Autodesk Inventor part; units mm, degrees
note: some values were not read from the file. Chosen so that the rebuilt part matches the saved one: direction of "Hole2".
(part 9 of 20)
  ellipse E68 centre (-104.430172, -37.80624) end of major axis (-105.229069, -37.764253) minor radius 0.002573 (-104.767308, -37.786185) -> (-104.757911, -37.791366) ccw
  line L116 (-105.229069, -37.764253) -> (-105.124102, -35.76702)
  line L117 (-102.853693, -35.883206) -> (-102.767428, -34.241823)
  line L118 (-103.727851, -35.778425) -> (-103.715482, -35.543073)
  ellipse E69 centre (-104.430172, -37.80624) end of major axis (-104.929483, -37.779998) minor radius 0.001608 (-104.765064, -37.787445) -> (-104.760245, -37.790101) ccw
  line L119 (-91.805643, -35.801391) -> (-92.357488, -33.197777)
  ellipse E70 centre (-90.362382, -35.950654) end of major axis (-88.992808, -35.660368) minor radius 0.211294 (-90.910001, -35.866075) -> (-90.933885, -35.8727) ccw
  line L120 (-90.98715, -35.502085) -> (-90.910001, -35.866075)
  line L121 (-91.937822, -36.388821) -> (-91.841267, -36.339714)
  line L122 (-90.910001, -35.866075) -> (-90.833464, -35.827148)
  line L123 (-91.937822, -36.388821) -> (-90.397989, -36.081252)
  ellipse E71 centre (-90.362382, -35.950654) end of major axis (-89.579768, -35.784776) minor radius 0.120739 (-90.397989, -36.081252) -> (-89.740826, -35.747021) ccw
  line L124 (-89.740826, -35.747021) -> (-90.657006, -35.748201)
  line L125 (-91.73285, -37.355883) -> (-91.937822, -36.388821)
  ellipse E72 centre (-89.952438, -37.884777) end of major axis (-90.735052, -38.050655) minor radius 0.120739 (-90.64361, -38.085759) -> (-89.235774, -37.786185) ccw
  line L126 (-89.578101, -35.792644) -> (-89.579768, -35.784776)
  line L127 (-91.937822, -36.388821) -> (-92.608968, -33.222344)
  line L128 (-91.73285, -37.355883) -> (-92.054619, -37.098206)
  ellipse E73 centre (-91.737472, -36.936906) end of major axis (-92.531076, -36.371583) minor radius 0.319988 (-92.547253, -36.492324) -> (-92.054619, -37.098206) ccw
  line L129 (-92.547253, -36.492324) -> (-93.874248, -30.231533)
  line L130 (-91.73285, -37.355883) -> (-90.193017, -37.048314)
  line L131 (-89.325137, -35.77526) -> (-89.388482, -35.213586)
  line L132 (-88.451238, -35.605729) -> (-88.440782, -35.698444)
  line L133 (-88.870762, -35.923384) -> (-88.001691, -35.82361)
  ellipse E74 centre (-87.925465, -35.832087) end of major axis (-87.130505, -35.742432) minor radius 0.01704 (-87.143191, -35.740852) -> (-88.001691, -35.82361) ccw
  ellipse E75 centre (-87.70138, -37.819037) end of major axis (-88.496341, -37.908691) minor radius 0.01704 (-86.979081, -37.730452) -> (-88.427677, -37.893938) ccw
  line L134 (-89.589644, -35.734525) -> (-89.646842, -35.227355)
  ellipse E76 centre (-89.482855, -22.022782) end of major axis (-87.406021, -21.788561) minor radius 0.044517 (-87.474249, -21.78497) -> (-87.899556, -21.815311) ccw
  ellipse E77 centre (-89.382017, -22.91691) end of major axis (-87.305183, -22.682688) minor radius 0.044517 (-87.376049, -22.679181) -> (-87.795125, -22.709125) ccw
  ellipse E78 centre (-87.813423, -36.825562) end of major axis (-88.608383, -36.915216) minor radius 0.01704 (-87.889648, -36.817085) -> (-88.582568, -36.90793) ccw
  line L135 (-88.81819, -36.923686) -> (-87.889648, -36.817085)
  ellipse E79 centre (-87.70138, -37.819037) end of major axis (-88.198231, -37.875071) minor radius 0.01065 (-87.22685, -37.762368) -> (-88.190637, -37.872322) ccw
  line L136 (-95.422117, -34.951561) -> (-95.372421, -34.494843)
  line L137 (-93.334624, -36.847285) -> (-94.485298, -36.84101)
  line L138 (-94.326748, -37.421303) -> (-93.014694, -37.428457)
  line L139 (-93.014694, -37.428457) -> (-92.908579, -37.255208)
  ellipse E80 centre (-93.582228, -37.251534) end of major axis (-92.87059, -37.067245) minor radius 0.371687 (-93.186534, -36.858933) -> (-93.334624, -36.847285) ccw
  ellipse E81 centre (-93.582228, -37.251534) end of major axis (-92.87059, -37.067245) minor radius 0.371687 (-92.908579, -37.255208) -> (-92.903906, -37.247372) ccw
  ellipse E82 centre (-94.728774, -37.966559) end of major axis (-93.933469, -38.053098) minor radius 0.273562 (-94.113945, -38.200163) -> (-93.998225, -38.145751) ccw
  line L140 (-98.417199, -34.951561) -> (-98.466895, -34.494843)
  ellipse E83 centre (-100.277081, -37.276138) end of major axis (-99.56931, -37.369327) minor radius 0.400382 (-100.444305, -36.869727) -> (-100.966797, -37.309126) ccw
  line L141 (-100.985403, -37.237624) -> (-101.000691, -37.09713)
  line L142 (-99.513466, -36.825206) -> (-100.444305, -36.869727)
  line L143 (-100.966797, -37.309126) -> (-100.895129, -37.483302)
  line L144 (-100.895129, -37.483302) -> (-99.67736, -37.425058)
  ellipse E84 centre (-99.274308, -37.966559) end of major axis (-100.069614, -38.053098) minor radius 0.273562 (-100.004857, -38.145751) -> (-99.889137, -38.200163) ccw
  ellipse E85 centre (-106.077617, -35.832087) end of major axis (-106.872577, -35.742432) minor radius 0.01704 (-106.083328, -35.814295) -> (-106.859892, -35.740852) ccw
  line L145 (-106.083328, -35.814295) -> (-105.132213, -35.921364)
  ellipse E86 centre (-106.301702, -37.819037) end of major axis (-107.096662, -37.729383) minor radius 0.01704 (-105.575405, -37.893938) -> (-107.024001, -37.730452) ccw
  line L146 (-104.489789, -35.736592) -> (-104.431907, -35.22335)
  ellipse E87 centre (-104.520227, -22.022782) end of major axis (-106.597061, -21.788561) minor radius 0.044517 (-106.103527, -21.815311) -> (-106.597061, -21.788561) ccw
  ellipse E88 centre (-104.621065, -22.91691) end of major axis (-106.697899, -22.682688) minor radius 0.044517 (-106.207957, -22.709125) -> (-106.627033, -22.679181) ccw
  line L147 (-106.195371, -36.80777) -> (-105.184779, -36.921534)
  ellipse E89 centre (-106.189659, -36.825562) end of major axis (-105.394699, -36.915216) minor radius 0.01704 (-105.420514, -36.90793) -> (-106.195371, -36.80777) ccw
  ellipse E90 centre (-106.301702, -37.819037) end of major axis (-106.798552, -37.763003) minor radius 0.01065 (-105.858125, -37.873868) -> (-106.750481, -37.773047) ccw
  line L148 (-103.182559, -35.813202) -> (-104.167244, -35.750402)
  ellipse E91 centre (-103.6407, -35.950654) end of major axis (-104.423314, -35.784776) minor radius 0.120739 (-104.167244, -35.750402) -> (-103.745321, -36.051258) ccw
  line L149 (-103.745321, -36.051258) -> (-102.217715, -36.399788)
  line L150 (-102.217715, -36.399788) -> (-102.422687, -37.36685)
  ellipse E92 centre (-104.050644, -37.884777) end of major axis (-104.833258, -37.718899) minor radius 0.120739 (-104.767308, -37.786185) -> (-103.359472, -38.085759) ccw
  line L151 (-104.424982, -35.792644) -> (-104.423314, -35.784776)
  line L152 (-102.250485, -36.376421) -> (-102.217715, -36.399788)
  line L153 (-102.217715, -36.399788) -> (-101.541613, -33.209926)
  ellipse E93 centre (-102.284453, -36.9758) end of major axis (-101.472148, -36.416877) minor radius 0.235923 (-102.080832, -37.120994) -> (-101.472427, -36.509437) ccw
  line L154 (-101.404603, -36.200633) -> (-100.152123, -30.291408)
  line L155 (-102.080832, -37.120994) -> (-102.422687, -37.36685)
  line L156 (-103.950293, -37.01832) -> (-102.422687, -37.36685)
  line L157 (-91.05411, -35.879044) -> (-91.076939, -35.444665)
  line L158 (-90.230803, -35.465481) -> (-90.215974, -35.747633)
  line L159 (-91.29938, -35.891986) -> (-89.730041, -35.809177)
  ellipse E94 centre (-89.677878, -35.809007) end of major axis (-88.87898, -35.76702) minor radius 0.002573 (-88.87898, -35.76702) -> (-89.730041, -35.809177) ccw
  line L160 (-91.296789, -35.941292) -> (-91.29938, -35.891986)
  ellipse E95 centre (-89.57291, -37.80624) end of major axis (-88.774013, -37.764253) minor radius 0.002573 (-89.245172, -37.791366) -> (-89.235774, -37.786185) ccw
  line L161 (-88.774013, -37.764253) -> (-88.87898, -35.76702)
  line L162 (-89.970222, -35.743864) -> (-89.985769, -35.448055)
  line L163 (-91.29938, -35.891986) -> (-91.385523, -34.252933)
  ellipse E96 centre (-89.57291, -37.80624) end of major axis (-89.073599, -37.779998) minor radius 0.001608 (-89.242837, -37.790101) -> (-89.238018, -37.787445) ccw
  line L164 (-88.579416, -35.694157) -> (-88.575478, -35.616282)
  line L165 (-87.658407, -35.518527) -> (-87.66871, -35.722319)
  line L166 (-88.844477, -35.685961) -> (-87.279448, -35.734356)
  ellipse E97 centre (-87.199512, -35.880709) end of major axis (-86.400533, -35.921103) minor radius 0.142983 (-86.400533, -35.921103) -> (-86.916832, -35.760642) ccw
  line L167 (-88.846734, -35.730605) -> (-88.844477, -35.685961)
  ellipse E98 centre (-87.298871, -37.845996) end of major axis (-86.499891, -37.88639) minor radius 0.142983 (-86.638988, -37.959011) -> (-86.979081, -37.730452) ccw
  line L168 (-86.499891, -37.88639) -> (-86.400533, -35.921103)
  line L169 (-87.403649, -35.730515) -> (-87.391234, -35.48496)
  line L170 (-88.844477, -35.685961) -> (-88.834557, -35.489748)
  line L171 (-88.754671, -33.90963) -> (-88.741991, -33.658819)
  ellipse E99 centre (-86.508969, -22.221966) end of major axis (-84.421635, -22.327495) minor radius 0.373543 (-84.421635, -22.327495) -> (-85.857037, -21.898574) ccw
  ellipse E100 centre (-86.553681, -23.106345) end of major axis (-84.466347, -23.211874) minor radius 0.373543 (-84.855794, -23.407002) -> (-85.889952, -22.784232) ccw
  line L172 (-84.421635, -22.327495) -> (-84.466347, -23.211874)
  ellipse E101 centre (-86.553681, -23.106345) end of major axis (-85.055594, -23.182084) minor radius 0.268093 (-85.19814, -23.286981) -> (-87.773888, -22.890892) ccw
  ellipse E102 centre (-87.298871, -37.845996) end of major axis (-86.799509, -37.871242) minor radius 0.089364 (-87.113287, -37.938145) -> (-87.283323, -37.757325) ccw
  line L173 (-92.998906, -37.402681) -> (-92.513899, -37.499993)
  line L174 (-92.513899, -37.499993) -> (-92.504619, -37.487523)
  ellipse E103 centre (-94.353837, -37.924209) end of major axis (-93.580574, -38.129305) minor radius 0.142054 (-93.998225, -38.145751) -> (-93.580574, -38.129305) ccw
  line L175 (-93.580574, -38.129305) -> (-93.394136, -37.426388)
  line L176 (-97.450158, -34.951561) -> (-97.421801, -34.494843)
  line L177 (-105.395973, -36.91016) -> (-105.187286, -36.969239)
  ellipse E104 centre (-105.630208, -36.995775) end of major axis (-106.398891, -36.77413) minor radius 0.14613 (-105.188594, -36.994129) -> (-105.420514, -36.90793) ccw
  ellipse E105 centre (-105.902602, -37.940463) end of major axis (-105.422175, -38.078991) minor radius 0.091331 (-105.743445, -38.074276) -> (-105.879328, -37.852122) ccw
  ellipse E106 centre (-105.902602, -37.940463) end of major axis (-105.133919, -38.162107) minor radius 0.14613 (-105.634452, -38.157355) -> (-105.575405, -37.893938) ccw
  line L178 (-105.133919, -38.162107) -> (-105.022824, -37.776821)
  ellipse E107 centre (-102.93673, -36.106911) end of major axis (-103.682535, -35.817472) minor radius 0.002457 (-103.628417, -35.837492) -> (-103.682535, -35.817472) ccw
  ellipse E108 centre (-102.93673, -36.106911) end of major axis (-102.190924, -36.39635) minor radius 0.002457 (-103.612298, -35.843617) -> (-103.614549, -35.842761) ccw
  line L179 (-101.551416, -36.641447) -> (-101.540632, -36.645629)
  line L180 (-101.540632, -36.645629) -> (-101.902428, -37.577881)
  ellipse E109 centre (-103.660323, -37.971415) end of major axis (-102.914518, -38.260854) minor radius 0.002457 (-103.369821, -38.086582) -> (-103.359472, -38.085759) ccw
  line L181 (-103.68619, -35.82689) -> (-103.682535, -35.817472)
  line L182 (-102.914518, -38.260854) -> (-102.55578, -37.336484)
  line L183 (-101.540632, -36.645629) -> (-101.524884, -36.605051)
  line L184 (-101.452389, -36.418253) -> (-99.538445, -31.486535)
  ellipse E110 centre (-101.752662, -37.31671) end of major axis (-100.860337, -36.923935) minor radius 0.168714 (-101.530862, -37.400618) -> (-100.861799, -36.955978) ccw
  line L185 (-100.861799, -36.955978) -> (-99.208221, -32.695154)
  line L186 (-101.530862, -37.400618) -> (-101.902428, -37.577881)
  line L187 (-101.902428, -37.577881) -> (-102.517352, -37.345251)
  line L188 (-102.480897, -37.353569) -> (-101.902428, -37.577881)
  ellipse E111 centre (-103.660323, -37.971415) end of major axis (-103.194195, -38.152314) minor radius 0.001536 (-103.367332, -38.086401) -> (-103.361886, -38.085968) ccw
  line L189 (-91.613539, -36.134298) -> (-90.335363, -35.889978)
  ellipse E112 centre (-90.284268, -35.882488) end of major axis (-89.498467, -35.732431) minor radius 0.002231 (-90.135583, -35.851865) -> (-90.335363, -35.889978) ccw
  ellipse E113 centre (-90.284268, -35.882488) end of major axis (-89.498467, -35.732431) minor radius 0.002231 (-89.498467, -35.732431) -> (-89.980553, -35.822396) ccw
  line L190 (-89.497225, -35.738934) -> (-89.498467, -35.732431)
  line L191 (-88.873766, -35.866229) -> (-87.933724, -35.761265)
  ellipse E114 centre (-89.104953, -23.113274) end of major axis (-87.612095, -22.967065) minor radius 0.24157 (-87.677538, -22.90597) -> (-87.775629, -22.875994) ccw
  ellipse E115 centre (-89.104953, -23.113274) end of major axis (-87.024905, -22.909556) minor radius 0.336587 (-87.098371, -22.83267) -> (-87.104345, -22.829762) ccw
  ellipse E116 centre (-87.66195, -37.846982) end of major axis (-88.15957, -37.895718) minor radius 0.080523 (-88.095363, -37.848555) -> (-88.145676, -37.874094) ccw
  ellipse E117 centre (-87.66195, -37.846982) end of major axis (-87.164331, -37.798246) minor radius 0.080523 (-87.174632, -37.784081) -> (-87.288761, -37.757867) ccw
  ellipse E118 centre (-103.712607, -35.91066) end of major axis (-102.927191, -36.062721) minor radius 0.086818 (-103.766394, -35.812171) -> (-104.360228, -35.736765) ccw
  line L192 (-103.766394, -35.812171) -> (-103.588186, -35.844875)
  line L193 (-91.006251, -36.071199) -> (-90.764705, -35.999517)
  ellipse E119 centre (-90.71868, -35.988107) end of major axis (-89.951703, -35.76063) minor radius 0.002152 (-90.57202, -35.942407) -> (-90.764705, -35.999517) ccw
  ellipse E120 centre (-90.71868, -35.988107) end of major axis (-89.951703, -35.76063) minor radius 0.002152 (-90.500776, -35.921328) -> (-90.503346, -35.922088) ccw
  ellipse E121 centre (-90.71868, -35.988107) end of major axis (-89.951703, -35.76063) minor radius 0.002152 (-89.952246, -35.760708) -> (-90.205619, -35.834272) ccw
  line L194 (-91.987497, -37.405497) -> (-92.086263, -37.07249)
  line L195 (-94.014167, -29.871815) -> (-94.02426, -29.874754)
  line L196 (-93.270796, -33.078635) -> (-94.118611, -30.22008)
  line L197 (-91.976236, -37.402218) -> (-91.987497, -37.405497)
  line L198 (-91.987497, -37.405497) -> (-92.05118, -37.365553)
  line L199 (-91.987497, -37.405497) -> (-91.756499, -37.336945)
  line L200 (-88.415292, -35.841908) -> (-88.397731, -35.838079)
  ellipse E122 centre (-88.323123, -35.953616) end of major axis (-87.539825, -35.791) minor radius 0.128538 (-88.161995, -35.792662) -> (-88.397731, -35.838079) ccw
  line L201 (-88.817348, -36.939713) -> (-88.754142, -36.925932)
  ellipse E123 centre (-87.921864, -37.88642) end of major axis (-88.411426, -37.988055) minor radius 0.080336 (-88.12131, -37.851814) -> (-88.276833, -38.014639) ccw
  ellipse E124 centre (-106.609775, -35.858739) end of major axis (-107.409757, -35.864011) minor radius 0.125799 (-106.589584, -35.732848) -> (-107.409757, -35.864011) ccw
  line L202 (-106.589584, -35.732848) -> (-105.874946, -35.731093)
  line L203 (-105.036889, -35.729035) -> (-105.015254, -35.728981)
  line L204 (-105.015254, -35.728981) -> (-105.015061, -35.758236)
  ellipse E125 centre (-106.59676, -37.833815) end of major axis (-107.396743, -37.839086) minor radius 0.125799 (-106.311855, -37.714431) -> (-106.576569, -37.707924) ccw
  line L205 (-105.015254, -35.728981) -> (-105.018797, -35.191274)
  line L206 (-105.025415, -34.186857) -> (-105.028812, -33.671406)
  ellipse E126 centre (-106.700226, -22.131966) end of major axis (-108.790181, -22.145737) minor radius 0.328649 (-106.862517, -21.805345) -> (-107.891271, -21.869557) ccw
  ellipse E127 centre (-106.69437, -23.02075) end of major axis (-108.784324, -23.034521) minor radius 0.328649 (-106.93899, -22.695925) -> (-107.877588, -22.757441) ccw
  ellipse E128 centre (-106.69437, -23.02075) end of major axis (-108.194337, -23.030633) minor radius 0.235872 (-106.217877, -22.794028) -> (-108.191997, -23.043547) ccw
  ellipse E129 centre (-106.59676, -37.833815) end of major axis (-107.096749, -37.837109) minor radius 0.078624 (-106.71236, -37.758062) -> (-106.891764, -37.899192) ccw
  ellipse E130 centre (-104.183501, -35.818698) end of major axis (-104.980671, -35.751457) minor radius 0.002201 (-104.267264, -35.809437) -> (-104.980671, -35.751457) ccw
  line L207 (-104.981419, -35.760336) -> (-104.980671, -35.751457)
  line L208 (-91.61255, -36.134109) -> (-92.161706, -33.174903)
  line L209 (-91.833694, -36.261711) -> (-91.607996, -36.175948)
  line L210 (-91.833694, -36.261711) -> (-90.286036, -35.982923)
  ellipse E131 centre (-90.257477, -35.898912) end of major axis (-89.470906, -35.752944) minor radius 0.077504 (-90.286036, -35.982923) -> (-89.630523, -35.736086) ccw
  ellipse E132 centre (-90.257477, -35.898912) end of major axis (-91.044047, -36.044881) minor radius 0.077504 (-89.632187, -35.736173) -> (-89.637416, -35.736455) ccw
  line L211 (-89.637416, -35.736455) -> (-89.681705, -35.738912)
  line L212 (-91.827408, -36.295579) -> (-91.833694, -36.261711)
  line L213 (-89.464627, -35.786781) -> (-89.470906, -35.752944)
  line L214 (-91.833694, -36.261711) -> (-92.093462, -34.861913)
  line L215 (-89.25094, -35.769186) -> (-89.305654, -35.209109)
  line L216 (-88.872594, -35.888539) -> (-87.92125, -35.79153)
  ellipse E133 centre (-87.858242, -35.831451) end of major axis (-87.062032, -35.753669) minor radius 0.045982 (-87.119951, -35.742267) -> (-87.92125, -35.79153) ccw
  line L217 (-89.505008, -35.733389) -> (-89.554918, -35.222487)
  ellipse E134 centre (-89.207472, -22.020177) end of major axis (-87.127374, -21.816972) minor radius 0.120129 (-87.140565, -21.805345) -> (-87.901453, -21.799074) ccw
  ellipse E135 centre (-89.120111, -22.914432) end of major axis (-87.040013, -22.711227) minor radius 0.120129 (-87.064092, -22.695925) -> (-87.308637, -22.678729) ccw
  ellipse E136 centre (-89.120111, -22.914432) end of major axis (-87.627218, -22.768591) minor radius 0.086217 (-87.781875, -22.822534) -> (-87.790867, -22.745575) ccw
  ellipse E137 centre (-87.664108, -37.818684) end of major axis (-87.166477, -37.77007) minor radius 0.028739 (-87.20767, -37.762739) -> (-87.224132, -37.762354) ccw
  line L218 (-104.713483, -35.208237) -> (-104.768154, -35.767882)
  ellipse E138 centre (-106.144841, -35.831451) end of major axis (-106.94105, -35.753669) minor radius 0.045982 (-106.128174, -35.786883) -> (-106.883131, -35.742267) ccw
  line L219 (-106.128174, -35.786883) -> (-105.130316, -35.885252)
  ellipse E139 centre (-104.795611, -22.020177) end of major axis (-106.875708, -21.816972) minor radius 0.120129 (-106.101629, -21.799074) -> (-106.862517, -21.805345) ccw
  ellipse E140 centre (-104.882971, -22.914432) end of major axis (-106.963069, -22.711227) minor radius 0.120129 (-106.694445, -22.678729) -> (-106.93899, -22.695925) ccw
  ellipse E141 centre (-104.882971, -22.914432) end of major axis (-106.375864, -22.768591) minor radius 0.086217 (-106.212215, -22.745575) -> (-106.221207, -22.822534) ccw
  ellipse E142 centre (-106.338974, -37.818684) end of major axis (-105.841343, -37.867298) minor radius 0.028739 (-105.860305, -37.873186) -> (-105.881624, -37.851833) ccw
  ellipse E143 centre (-106.338974, -37.818684) end of major axis (-106.836605, -37.77007) minor radius 0.028739 (-106.618921, -37.767554) -> (-106.813201, -37.781264) ccw
  line L220 (-101.888103, -33.169443) -> (-102.432316, -36.102017)
  ellipse E144 centre (-103.745605, -35.898912) end of major axis (-104.532176, -35.752944) minor radius 0.077504 (-104.360228, -35.736765) -> (-103.821607, -35.963391) ccw
  line L221 (-103.821607, -35.963391) -> (-102.343144, -36.249471)
  line L222 (-104.538455, -35.786781) -> (-104.532176, -35.752944)
  line L223 (-91.426481, -35.952249) -> (-89.859121, -35.819828)
  ellipse E145 centre (-89.819581, -35.818698) end of major axis (-89.022412, -35.751457) minor radius 0.002201 (-89.737454, -35.809574) -> (-89.859121, -35.819828) ccw
  ellipse E146 centre (-89.819581, -35.818698) end of major axis (-89.022412, -35.751457) minor radius 0.002201 (-89.022412, -35.751457) -> (-89.737257, -35.809558) ccw
  line L224 (-91.414337, -36.096221) -> (-91.426481, -35.952249)
  line L225 (-89.021663, -35.760336) -> (-89.022412, -35.751457)
  line L226 (-91.426481, -35.952249) -> (-91.57069, -34.242604)
  line L227 (-91.663147, -33.146486) -> (-91.665639, -33.116944)
  line L228 (-87.900207, -35.546912) -> (-87.901315, -35.715126)
  line L229 (-89.02939, -35.743523) -> (-87.460048, -35.732948)
  ellipse E147 centre (-87.393307, -35.858739) end of major axis (-86.593325, -35.864011) minor radius 0.125799 (-86.959772, -35.755799) -> (-87.460048, -35.732948) ccw
  line L230 (-89.029444, -35.751758) -> (-89.02939, -35.743523)
  line L231 (-89.02939, -35.743523) -> (-89.025766, -35.193642)
  line L232 (-89.019145, -34.188784) -> (-89.013946, -33.399804)
  ellipse E148 centre (-87.302856, -22.131966) end of major axis (-89.392811, -22.118194) minor radius 0.328649 (-86.111811, -21.869557) -> (-87.140565, -21.805345) ccw
  ellipse E149 centre (-87.308712, -23.02075) end of major axis (-89.398667, -23.006978) minor radius 0.328649 (-86.125494, -22.757441) -> (-87.064092, -22.695925) ccw
  ellipse E150 centre (-87.308712, -23.02075) end of major axis (-85.808745, -23.030633) minor radius 0.235872 (-85.826668, -23.06663) -> (-87.785206, -22.794028) ccw
  ellipse E151 centre (-87.399815, -36.846277) end of major axis (-88.199797, -36.841005) minor radius 0.125799 (-87.466556, -36.720485) -> (-87.787907, -36.733777) ccw
  ellipse E152 centre (-87.406322, -37.833815) end of major axis (-86.906333, -37.837109) minor radius 0.078624 (-87.053751, -37.780331) -> (-87.290722, -37.758062) ccw
  line L233 (-105.197035, -36.931057) -> (-105.185407, -36.933478)
  ellipse E153 centre (-106.081218, -37.88642) end of major axis (-105.591656, -37.988055) minor radius 0.080336 (-105.726249, -38.014639) -> (-105.881772, -37.851814) ccw
  ellipse E154 centre (-103.284402, -35.988107) end of major axis (-104.051379, -35.76063) minor radius 0.002152 (-103.798778, -35.833885) -> (-104.050836, -35.760708) ccw
  line L234 (-100.487604, -31.874214) -> (-99.938432, -30.022584)
  line L235 (-99.979109, -29.873706) -> (-99.988585, -29.870969)
  ellipse E155 centre (-89.105164, -33.361974) end of major axis (-88.264589, -33.157869) minor radius 0.148059 (-89.226144, -33.239793) -> (-89.296203, -33.258672) ccw
  ellipse E156 centre (-89.105164, -33.361974) end of major axis (-88.264589, -33.157869) minor radius 0.148059 (-89.03551, -33.193878) -> (-89.08253, -33.204474) ccw
  ellipse E157 centre (-106.775628, -32.550102) end of major axis (-106.318773, -32.538591) minor radius 0.076505 (-106.395552, -32.498331) -> (-106.94859, -32.483506) ccw
  ellipse E158 centre (-106.775628, -32.550102) end of major axis (-107.640354, -32.571891) minor radius 0.144806 (-106.274061, -32.419823) -> (-107.482519, -32.650845) ccw
  ellipse E159 centre (-106.800462, -31.564527) end of major axis (-107.665187, -31.586315) minor radius 0.144806 (-106.582905, -31.419007) -> (-107.665187, -31.586315) ccw
  line L236 (-107.665187, -31.586315) -> (-107.640354, -32.571891)
  ellipse E160 centre (-104.059443, -33.289753) end of major axis (-104.922235, -33.227976) minor radius 0.002538 (-103.961875, -33.294212) -> (-104.706167, -33.245131) ccw
  line L237 (-104.892906, -32.818372) -> (-104.922235, -33.227976)
  ellipse E161 centre (-88.125069, -33.582649) end of major axis (-88.985365, -33.672736) minor radius 0.036963 (-87.26884, -33.496765) -> (-88.966084, -33.678381) ccw
  ellipse E162 centre (-88.229122, -32.588995) end of major axis (-87.368826, -32.498908) minor radius 0.036963 (-87.368826, -32.498908) -> (-88.608725, -32.595322) ccw
  line L238 (-87.368826, -32.498908) -> (-87.264773, -33.492561)
  line L239 (-89.075259, -32.814293) -> (-88.985365, -33.672736)
  ellipse E163 centre (-105.878013, -33.582649) end of major axis (-106.738309, -33.492561) minor radius 0.036963 (-105.017724, -33.672797) -> (-106.734242, -33.496765) ccw
  ellipse E164 centre (-105.77396, -32.588995) end of major axis (-106.634256, -32.498908) minor radius 0.036963 (-105.394357, -32.595322) -> (-106.634256, -32.498908) ccw
  line L240 (-104.927823, -32.814293) -> (-105.017717, -33.672736)
  line L241 (-106.634256, -32.498908) -> (-106.738309, -33.492561)
  ellipse E165 centre (-89.943639, -33.289753) end of major axis (-89.080848, -33.227976) minor radius 0.002538 (-89.296915, -33.245131) -> (-90.041208, -33.294212) ccw
  line L242 (-89.110176, -32.818372) -> (-89.080848, -33.227976)
  ellipse E166 centre (-87.227454, -32.550102) end of major axis (-86.770599, -32.561614) minor radius 0.076505 (-87.054492, -32.483506) -> (-87.60753, -32.498331) ccw
  ellipse E167 centre (-87.227454, -32.550102) end of major axis (-86.362728, -32.571891) minor radius 0.144806 (-86.520563, -32.650845) -> (-87.729021, -32.419823) ccw
  ellipse E168 centre (-87.20262, -31.564527) end of major axis (-86.337895, -31.586315) minor radius 0.144806 (-86.337895, -31.586315) -> (-87.420178, -31.419007) ccw
  line L243 (-86.337895, -31.586315) -> (-86.362728, -32.571891)
  ellipse E169 centre (-90.540377, -35.326807) end of major axis (-90.986594, -35.425498) minor radius 0.001467 (-90.21271, -35.253317) -> (-90.974981, -35.423269) ccw
  ellipse E170 centre (-90.540377, -35.326807) end of major axis (-89.695788, -35.140008) minor radius 0.002777 (-90.129742, -35.233502) -> (-91.220763, -35.475602) ccw
  ellipse E171 centre (-90.756329, -34.350408) end of major axis (-89.91174, -34.163609) minor radius 0.002777 (-90.029814, -34.188275) -> (-91.336758, -34.476715) ccw
  line L244 (-87.22699, -34.340899) -> (-87.21537, -34.443342)
  line L245 (-106.776092, -34.340899) -> (-106.787712, -34.443342)
  ellipse E172 centre (-103.462705, -35.326807) end of major axis (-103.016489, -35.425498) minor radius 0.001467 (-103.028101, -35.423269) -> (-103.790372, -35.253317) ccw
  ellipse E173 centre (-103.462705, -35.326807) end of major axis (-102.618116, -35.513606) minor radius 0.002777 (-102.931279, -35.442132) -> (-103.87334, -35.233502) ccw
  ellipse E174 centre (-103.246753, -34.350408) end of major axis (-102.402164, -34.537208) minor radius 0.002777 (-102.848282, -34.43603) -> (-103.973268, -34.188275) ccw
  ellipse E175 centre (-90.531336, -35.452572) end of major axis (-90.085488, -35.352233) minor radius 0.077418 (-90.331924, -35.47998) -> (-90.934549, -35.506634) ccw
  ellipse E176 centre (-90.531336, -35.452572) end of major axis (-89.687443, -35.262652) minor radius 0.146534 (-90.989348, -35.426445) -> (-91.076298, -35.456866) ccw
  ellipse E177 centre (-90.531336, -35.452572) end of major axis (-89.687443, -35.262652) minor radius 0.146534 (-90.077265, -35.480008) -> (-89.728387, -35.230805) ccw
  line L246 (-89.694834, -35.229811) -> (-89.687443, -35.262652)
  ellipse E178 centre (-103.471746, -35.452572) end of major axis (-103.917595, -35.352233) minor radius 0.077418 (-103.063019, -35.509988) -> (-103.584595, -35.504657) ccw
  ellipse E179 centre (-103.471746, -35.452572) end of major axis (-102.627853, -35.642491) minor radius 0.146534 (-102.991901, -35.433802) -> (-103.013734, -35.426445) ccw
  ellipse E180 centre (-103.471746, -35.452572) end of major axis (-104.315639, -35.262652) minor radius 0.146534 (-104.274695, -35.230805) -> (-103.715173, -35.543157) ccw
  line L247 (-104.308248, -35.229811) -> (-104.315639, -35.262652)
  ellipse E181 centre (-91.765344, -34.3058) end of major axis (-90.958942, -33.992845) minor radius 0.002657 (-91.591538, -34.235566) -> (-91.939792, -34.370719) ccw
  ellipse E182 centre (-92.12714, -33.373548) end of major axis (-91.320738, -33.060593) minor radius 0.002657 (-91.818749, -33.251234) -> (-92.12549, -33.370058) ccw
  ellipse E183 centre (-89.187606, -34.170212) end of major axis (-88.356467, -33.930559) minor radius 0.158003 (-89.053067, -33.970764) -> (-89.2559, -34.025536) ccw
  ellipse E184 centre (-89.187606, -34.170212) end of major axis (-88.356467, -33.930559) minor radius 0.158003 (-88.661989, -33.896794) -> (-88.999448, -33.957952) ccw
  ellipse E185 centre (-106.881169, -34.34582) end of major axis (-107.337586, -34.368895) minor radius 0.081679 (-106.653684, -34.263788) -> (-106.785186, -34.421074) ccw
  ellipse E186 centre (-106.881169, -34.34582) end of major axis (-107.745066, -34.389496) minor radius 0.1546 (-106.411022, -34.192948) -> (-106.797394, -34.495782) ccw
  ellipse E187 centre (-106.930848, -33.363177) end of major axis (-107.794745, -33.406853) minor radius 0.1546 (-106.707957, -33.202718) -> (-107.794745, -33.406853) ccw
  line L248 (-107.794745, -33.406853) -> (-107.745066, -34.389496)
  ellipse E188 centre (-104.294659, -35.227812) end of major axis (-104.751029, -35.203827) minor radius 0.00147 (-103.900176, -35.249285) -> (-104.066874, -35.241059) ccw
  ellipse E189 centre (-104.294659, -35.227812) end of major axis (-105.158467, -35.182414) minor radius 0.002783 (-103.790217, -35.252062) -> (-104.308264, -35.229883) ccw
  ellipse E190 centre (-104.242175, -34.229196) end of major axis (-103.378367, -34.274594) minor radius 0.002783 (-103.499381, -34.266811) -> (-103.652652, -34.258142) ccw
  ellipse E191 centre (-104.242175, -34.229196) end of major axis (-105.105983, -34.183797) minor radius 0.002783 (-103.740115, -34.253314) -> (-105.105983, -34.183797) ccw
  line L249 (-105.105983, -34.183797) -> (-105.158467, -35.182414)
  ellipse E192 centre (-90.768637, -34.033937) end of major axis (-91.614838, -34.213292) minor radius 0.130549 (-91.614838, -34.213292) -> (-89.922435, -33.854582) ccw
  ellipse E193 centre (-90.973609, -33.066875) end of major axis (-91.81981, -33.246231) minor radius 0.130549 (-91.707464, -33.152207) -> (-90.169332, -32.94212) ccw
  line L250 (-90.117127, -32.936021) -> (-89.922435, -33.854582)
  line L251 (-91.81981, -33.246231) -> (-91.614838, -34.213292)
  ellipse E194 centre (-87.958966, -35.535038) end of major axis (-87.504845, -35.483823) minor radius 0.009734
  ellipse E195 centre (-87.958966, -35.535038) end of major axis (-88.818517, -35.631976) minor radius 0.018424 (-88.575538, -35.61746) -> (-88.802955, -35.63369) ccw
  ellipse E196 centre (-88.071008, -34.541562) end of major axis (-88.930559, -34.638501) minor radius 0.018424 (-87.211457, -34.444624) -> (-88.873888, -34.625447) ccw
  line L252 (-87.211457, -34.444624) -> (-87.099415, -35.438099)
  line L253 (-88.868999, -35.184353) -> (-88.818517, -35.631976)
  ellipse E197 centre (-106.044116, -35.535038) end of major axis (-106.498237, -35.483823) minor radius 0.009734
  ellipse E198 centre (-106.044116, -35.535038) end of major axis (-106.903667, -35.438099) minor radius 0.018424 (-105.187945, -35.629907) -> (-105.454272, -35.615015) ccw
  ellipse E199 centre (-105.932074, -34.541562) end of major axis (-106.791625, -34.444624) minor radius 0.018424 (-105.129194, -34.625447) -> (-106.791625, -34.444624) ccw
  line L254 (-106.791625, -34.444624) -> (-106.903667, -35.438099)
  ellipse E200 centre (-103.234445, -34.033937) end of major axis (-104.080647, -33.854582) minor radius 0.130549 (-104.080647, -33.854582) -> (-102.388244, -34.213292) ccw
  ellipse E201 centre (-103.029474, -33.066875) end of major axis (-103.875675, -32.88752) minor radius 0.130549 (-103.83375, -32.94212) -> (-102.214446, -33.199411) ccw
  line L255 (-102.183272, -33.246231) -> (-102.388244, -34.213292)
  line L256 (-103.885955, -32.936021) -> (-104.080647, -33.854582)
  ellipse E202 centre (-89.708423, -35.227812) end of major axis (-90.164793, -35.251797) minor radius 0.00147 (-89.936208, -35.241059) -> (-90.102906, -35.249285) ccw
  ellipse E203 centre (-89.708423, -35.227812) end of major axis (-88.844615, -35.182414) minor radius 0.002783 (-89.694818, -35.229883) -> (-90.212865, -35.252062) ccw
  ellipse E204 centre (-89.760907, -34.229196) end of major axis (-88.897099, -34.183797) minor radius 0.002783 (-90.35043, -34.258142) -> (-90.503701, -34.266811) ccw
  ellipse E205 centre (-89.760907, -34.229196) end of major axis (-88.897099, -34.183797) minor radius 0.002783 (-88.897099, -34.183797) -> (-90.262967, -34.253314) ccw
  line L257 (-88.897099, -34.183797) -> (-88.844615, -35.182414)
  ellipse E206 centre (-87.121913, -34.34582) end of major axis (-86.665496, -34.368895) minor radius 0.081679 (-87.217896, -34.421074) -> (-87.349398, -34.263788) ccw
  ellipse E207 centre (-87.121913, -34.34582) end of major axis (-86.258016, -34.389496) minor radius 0.1546 (-87.205688, -34.495782) -> (-87.59206, -34.192948) ccw
  ellipse E208 centre (-87.072234, -33.363177) end of major axis (-86.208337, -33.406853) minor radius 0.1546 (-86.208337, -33.406853) -> (-87.295125, -33.202718) ccw
  line L258 (-86.208337, -33.406853) -> (-86.258016, -34.389496)
  ellipse E209 centre (-104.815476, -34.170212) end of major axis (-103.984337, -34.409866) minor radius 0.158003 (-104.747182, -34.025536) -> (-104.821673, -34.004282) ccw
  ellipse E210 centre (-102.237738, -34.3058) end of major axis (-101.431337, -34.618756) minor radius 0.002657 (-102.107817, -34.353408) -> (-102.241212, -34.301603) ccw
  ellipse E211 centre (-101.875942, -33.373548) end of major axis (-101.06954, -33.686504) minor radius 0.002657 (-101.922125, -33.35278) -> (-102.110585, -33.279761) ccw
  ellipse E212 centre (-88.447058, -29.69633) end of major axis (-87.586074, -29.613075) minor radius 0.221488 (-87.866284, -29.479621) -> (-87.962372, -29.468679) ccw
  ellipse E213 centre (-105.556024, -29.69633) end of major axis (-104.69504, -29.779584) minor radius 0.221488 (-106.04071, -29.468679) -> (-106.136798, -29.479621) ccw
  ellipse E214 centre (-106.643749, -30.702805) end of major axis (-106.186759, -30.699794) minor radius 0.071862 (-106.506157, -30.633392) -> (-106.83643, -30.638879) ccw
  ellipse E215 centre (-106.643749, -30.702805) end of major axis (-107.508731, -30.708505) minor radius 0.13602 (-106.499745, -30.567755) -> (-107.507413, -30.700849) ccw
  ellipse E216 centre (-106.650257, -29.715267) end of major axis (-107.515238, -29.720967) minor radius 0.13602 (-106.054787, -29.612782) -> (-107.510285, -29.706259) ccw
  ellipse E217 centre (-88.270291, -31.613547) end of major axis (-87.815456, -31.569114) minor radius 0.026267 (-87.817786, -31.572161) -> (-87.818372, -31.566559) ccw
  ellipse E218 centre (-88.270291, -31.613547) end of major axis (-87.409389, -31.529445) minor radius 0.049718 (-87.419159, -31.538187) -> (-88.455273, -31.582771) ccw
  ellipse E219 centre (-88.367357, -30.619931) end of major axis (-87.506456, -30.535829) minor radius 0.049718 (-87.506456, -30.535829) -> (-88.300826, -30.563648) ccw
  line L259 (-87.506456, -30.535829) -> (-87.409389, -31.529445)
  ellipse E220 centre (-105.732792, -31.613547) end of major axis (-106.187626, -31.569114) minor radius 0.026267 (-106.18471, -31.566559) -> (-106.185296, -31.572161) ccw
  ellipse E221 centre (-105.732792, -31.613547) end of major axis (-106.593693, -31.529445) minor radius 0.049718 (-105.547809, -31.582771) -> (-106.583923, -31.538187) ccw
  ellipse E222 centre (-105.635725, -30.619931) end of major axis (-106.496626, -30.535829) minor radius 0.049718 (-105.702256, -30.563648) -> (-106.496626, -30.535829) ccw
  line L260 (-106.496626, -30.535829) -> (-106.593693, -31.529445)
  ellipse E223 centre (-87.359333, -30.702805) end of major axis (-86.902343, -30.705816) minor radius 0.071862 (-87.166652, -30.638879) -> (-87.496925, -30.633392) ccw
  ellipse E224 centre (-87.359333, -30.702805) end of major axis (-86.494351, -30.708505) minor radius 0.13602 (-86.495669, -30.700849) -> (-87.503337, -30.567755) ccw
  ellipse E225 centre (-87.352825, -29.715267) end of major axis (-86.487844, -29.720967) minor radius 0.13602 (-86.492797, -29.706259) -> (-87.948295, -29.612782) ccw
  ellipse E226 centre (-97.001541, 42.174038) end of major axis (-96.935625, 42.91435) minor radius 0.194882 (-96.796541, 42.395712) -> (-97.206541, 41.952364) ccw
  line L261 (-97.206541, 39.942706) -> (-97.206541, 41.952364)
  line L262 (-96.796541, 40.385469) -> (-96.796541, 42.395712)
  ellipse E227 centre (-94.867221, 42.174459) end of major axis (-94.724063, 42.928567) minor radius 0.195462 (-94.640129, 42.374917) -> (-94.91501, 42.704151) ccw
  line L263 (-97.350612, 20.408579) -> (-97.266479, 21.212717)
  line L264 (-94.801473, 40.832805) -> (-94.640129, 42.374917)
  ellipse E228 centre (-99.135861, 42.174459) end of major axis (-99.151958, 42.941861) minor radius 0.195482 (-99.110088, 42.925229) -> (-99.316567, 41.931565) ccw
  line L265 (-99.211438, 40.926751) -> (-99.316567, 41.931565)
  line L266 (-96.65247, 20.408579) -> (-96.736603, 21.212717)
  ellipse E229 centre (-97.001541, 40.164088) end of major axis (-96.935376, 40.901077) minor radius 0.194809 (-96.796541, 40.385469) -> (-97.206541, 39.942706) ccw
  line L267 (-97.206541, 23.407456) -> (-97.206541, 39.942706)
  line L268 (-96.796541, 23.407456) -> (-96.796541, 40.385469)
  ellipse E230 centre (-94.836069, 40.163952) end of major axis (-94.683838, 40.916276) minor radius 0.195466 (-94.60658, 40.361612) -> (-94.905112, 40.628679) ccw
  line L269 (-98.170114, 13.39451) -> (-97.350595, 20.408745)
  line L270 (-96.784649, 21.719606) -> (-94.60658, 40.361612)
  line L271 (-97.206541, 13.392657) -> (-97.206541, 19.897109)
  line L272 (-96.796541, 13.392657) -> (-96.796541, 19.897109)
  ellipse E231 centre (-99.167013, 40.163952) end of major axis (-99.192352, 40.931102) minor radius 0.195478 (-99.126999, 40.890944) -> (-99.344771, 39.918852) ccw
  line L273 (-97.218433, 21.719606) -> (-99.344771, 39.918852)
  line L274 (-95.832968, 13.39451) -> (-96.652487, 20.408745)
  ellipse E232 centre (-97.001541, 44.202145) end of major axis (-96.937663, 44.967042) minor radius 0.195472 (-96.796541, 44.425031) -> (-97.206541, 43.979259) ccw
  line L275 (-97.206541, 43.958231) -> (-97.206541, 43.979259)
  line L276 (-96.796541, 44.402011) -> (-96.796541, 44.425031)
  ellipse E233 centre (-97.001541, 44.180121) end of major axis (-96.935827, 44.923078) minor radius 0.19494 (-96.796541, 44.402011) -> (-97.206541, 43.958231) ccw
  line L277 (-97.206541, 41.952364) -> (-97.206541, 43.958231)
  line L278 (-96.796541, 42.395712) -> (-96.796541, 44.402011)
  ellipse E234 centre (-94.883491, 44.180946) end of major axis (-94.747705, 44.936403) minor radius 0.195467 (-94.658368, 44.383544) -> (-95.108613, 43.978347) ccw
  ellipse E235 centre (-97.802609, 13.384052) end of major axis (-97.598523, 13.364708) minor radius 0.000002 (-97.598523, 13.364708) -> (-97.844396, 13.388016) ccw
  line L279 (-97.266564, 21.211819) -> (-97.218424, 21.719697)
  line L280 (-96.796541, 26.17059) -> (-95.108613, 43.978347)
  line L281 (-97.598523, 13.364708) -> (-97.206541, 17.500147)
  line L282 (-94.799515, 42.894439) -> (-94.658368, 44.383544)
  ellipse E236 centre (-99.119591, 44.180946) end of major axis (-99.128191, 44.948458) minor radius 0.195476 (-98.936533, 44.42213) -> (-99.302649, 43.939761) ccw
  ellipse E237 centre (-96.200474, 13.384052) end of major axis (-96.404559, 13.364708) minor radius 0.000002 (-96.158686, 13.388016) -> (-96.404559, 13.364708) ccw
  line L283 (-96.404559, 13.364708) -> (-96.796541, 17.500147)
  line L284 (-99.205144, 42.911075) -> (-99.302649, 43.939761)
  line L285 (-96.736518, 21.211819) -> (-96.784658, 21.719697)
  line L286 (-97.206541, 26.17059) -> (-98.936533, 44.42213)
  line L287 (-106.053523, -29.351646) -> (-106.027815, -29.336686)
  line L288 (-106.111967, -29.231664) -> (-106.104839, -29.233236)
  line L289 (-106.138331, -29.247006) -> (-106.111967, -29.231664)
  line L290 (-106.111967, -29.231664) -> (-106.108873, -29.201754)
  line L291 (-107.71687, -29.199141) -> (-107.699561, -29.199949)
  line L292 (-107.699561, -29.199949) -> (-107.652162, -29.180108)
  line L293 (-107.548659, -29.136781) -> (-107.515543, -29.122918)
  line L294 (-107.344396, -29.051276) -> (-107.32025, -29.041168)
  line L295 (-107.513458, -29.032144) -> (-107.32025, -29.041168)
  line L296 (-107.595141, -29.066337) -> (-107.513458, -29.032144)
  line L297 (-107.32025, -29.041168) -> (-107.320281, -29.039923)
  line L298 (-107.513458, -29.032144) -> (-107.514882, -28.97563)
  line L299 (-107.56134, -27.131815) -> (-107.561349, -27.131462)
  line L300 (-107.614102, -25.03783) -> (-107.614727, -25.013015)
  line L301 (-106.949693, -28.980234) -> (-106.986799, -28.995767)
  line L302 (-106.950022, -28.967184) -> (-106.949693, -28.980234)
  line L303 (-106.949693, -28.980234) -> (-106.832242, -28.98572)
  line L304 (-106.682343, -28.992721) -> (-106.19817, -29.015335)
  line L305 (-87.766198, -29.062637) -> (-87.739288, -29.060377)
  line L306 (-87.495774, -29.039932) -> (-87.487045, -29.039199)
  line L307 (-87.23192, -28.975887) -> (-87.206533, -28.983077)
  line L308 (-87.291171, -28.980861) -> (-87.23192, -28.975887)
  line L309 (-87.23192, -28.975887) -> (-87.23145, -28.957217)
  line L310 (-86.811329, -28.933066) -> (-86.813684, -29.026553)
  line L311 (-86.637458, -29.011757) -> (-86.813684, -29.026553)
  line L312 (-86.536151, -24.991163) -> (-86.536612, -25.009428)
  line L313 (-86.589567, -27.111075) -> (-86.590101, -27.132279)
  line L314 (-86.635765, -28.944565) -> (-86.637458, -29.011757)
  line L315 (-86.813684, -29.026553) -> (-86.689811, -29.061637)
  line L316 (-86.407367, -29.141632) -> (-86.394387, -29.145308)
  line L317 (-86.637458, -29.011757) -> (-86.478971, -29.056645)
  line L318 (-86.328954, -29.231629) -> (-86.347433, -29.226395)
  line L319 (-87.87076, -29.0855) -> (-87.857905, -29.087812)
  line L320 (-107.651638, -29.305727) -> (-107.877176, -29.298097)
  line L321 (-107.965137, -29.336516) -> (-107.877176, -29.298097)
  line L322 (-107.649542, -29.347194) -> (-107.965137, -29.336516)
  line L323 (-107.965137, -29.336516) -> (-107.967507, -29.289635)
  line L324 (-108.174904, -29.244657) -> (-107.984499, -29.251099)
  line L325 (-108.177681, -29.189727) -> (-108.174904, -29.244657)
  line L326 (-107.984499, -29.251099) -> (-107.578204, -29.073637)
  line L327 (-107.768609, -29.067195) -> (-107.578204, -29.073637)
  line L328 (-108.174904, -29.244657) -> (-107.768609, -29.067195)
  line L329 (-107.578204, -29.073637) -> (-107.578528, -29.067217)
  line L330 (-107.768609, -29.067195) -> (-107.769087, -29.057743)
  line L331 (-107.401022, -24.998287) -> (-107.399485, -25.028691)
  line L332 (-87.081317, -29.049926) -> (-87.07824, -29.049749)
  line L333 (-86.862818, -29.037365) -> (-86.804062, -29.033988)
  line L334 (-86.911174, -28.996436) -> (-86.804062, -29.033988)
  line L335 (-86.966905, -28.99964) -> (-86.911174, -28.996436)
  line L336 (-86.804062, -29.033988) -> (-86.803828, -29.029344)
  line L337 (-86.911174, -28.996436) -> (-86.908251, -28.938638)
  line L338 (-86.815967, -27.113283) -> (-86.815367, -27.101409)
  line L339 (-86.502731, -29.058428) -> (-86.502935, -29.062467)
  line L340 (-86.322607, -29.052101) -> (-86.502935, -29.062467)
  line L341 (-86.321641, -29.033) -> (-86.322607, -29.052101)
  line L342 (-86.502935, -29.062467) -> (-86.008183, -29.235919)
  line L343 (-85.827855, -29.225553) -> (-86.008183, -29.235919)
  line L344 (-86.322607, -29.052101) -> (-85.827855, -29.225553)
  line L345 (-85.827855, -29.225553) -> (-85.825186, -29.172766)
  line L346 (-85.977776, -29.32367) -> (-86.084887, -29.286119)
  line L347 (-85.9753, -29.274707) -> (-85.977776, -29.32367)
  line L348 (-86.084887, -29.286119) -> (-86.351227, -29.301429)
  line L349 (-85.977776, -29.32367) -> (-86.353443, -29.345266)
  line L350 (-107.136673, -29.035333) -> (-107.069759, -29.013719)
  line L351 (-107.257831, -29.000237) -> (-107.069759, -29.013719)
  line L352 (-107.365563, -29.035036) -> (-107.257831, -29.000237)
  line L353 (-107.069759, -29.013719) -> (-107.070092, -28.963121)
  line L354 (-107.0823, -27.110527) -> (-107.085083, -26.688057)
  line L355 (-107.257831, -29.000237) -> (-107.258118, -28.95676)
  line L356 (-107.270341, -27.101744) -> (-107.270381, -27.09577)
  line L357 (-107.284201, -24.998388) -> (-107.284377, -24.971637)
  line L358 (-88.002732, -29.05554) -> (-87.277768, -28.995031)
  line L359 (-87.381982, -28.965692) -> (-87.277768, -28.995031)
  line L360 (-87.658022, -28.988732) -> (-87.381982, -28.965692)
  line L361 (-87.277768, -28.995031) -> (-87.277703, -28.985138)
  line L362 (-87.381982, -28.965692) -> (-87.381836, -28.943489)
  line L363 (-87.35564, -24.968034) -> (-87.355436, -24.937038)
  line L364 (-104.43454, -10.841377) -> (-105.429773, -10.737374)
  line L365 (-108.228231, -9.942207) -> (-105.377744, -10.240088)
  ellipse E238 centre (-106.075125, -10.167567) end of major axis (-108.561553, -9.907422) minor radius 0.000177 (-108.228231, -9.942207) -> (-108.561553, -9.907422) ccw
  line L366 (-108.759085, -11.795411) -> (-108.561553, -9.907422)
  line L367 (-88.573309, -10.737374) -> (-89.568542, -10.841377)
  line L368 (-88.625338, -10.240088) -> (-85.774851, -9.942207)
  ellipse E239 centre (-87.927957, -10.167567) end of major axis (-85.441529, -9.907422) minor radius 0.000177 (-85.441529, -9.907422) -> (-85.774851, -9.942207) ccw
  line L369 (-85.441529, -9.907422) -> (-85.243997, -11.795411)
  ellipse E240 centre (-105.801133, -14.657855) end of major axis (-106.049444, -14.628843) minor radius 0.000013
  ellipse E241 centre (-104.732688, -14.78272) end of major axis (-105.325555, -14.713451) minor radius 0.00003 (-105.27471, -14.71938) -> (-105.274713, -14.719404) ccw
  ellipse E242 centre (-108.221697, -14.375261) end of major axis (-107.431228, -14.467616) minor radius 0.000039 (-108.571176, -14.334395) -> (-108.571284, -14.334452) ccw
  line L370 (-105.274687, -14.719187) -> (-109.114843, -14.270857)
  ellipse E243 centre (-106.964533, -14.522155) end of major axis (-109.447642, -14.232037) minor radius 0.000126 (-109.107483, -14.271716) -> (-109.447599, -14.232041) ccw
  line L371 (-108.824724, -11.787747) -> (-105.978348, -12.120056)
  ellipse E244 centre (-106.674415, -12.039046) end of major axis (-109.157524, -11.748928) minor radius 0.000126 (-108.824724, -11.787747) -> (-109.157524, -11.748928) ccw
  line L372 (-109.447642, -14.232037) -> (-109.157524, -11.748928)
  ellipse E245 centre (-101.302686, -15.183571) end of major axis (-109.745258, -14.197169) minor radius 0.000429 (-109.323636, -14.246565) -> (-108.571438, -14.334534) ccw
  line L373 (-105.04272, -12.732685) -> (-106.036372, -12.616678)
  ellipse E246 centre (-88.201949, -14.657855) end of major axis (-88.45026, -14.686867) minor radius 0.000013
  ellipse E247 centre (-89.270394, -14.78272) end of major axis (-88.677527, -14.713451) minor radius 0.00003 (-88.728369, -14.719404) -> (-88.728372, -14.71938) ccw
  ellipse E248 centre (-92.700396, -15.183571) end of major axis (-84.257824, -14.197169) minor radius 0.000429 (-85.431644, -14.334534) -> (-84.679446, -14.246565) ccw
  ellipse E249 centre (-87.038549, -14.522155) end of major axis (-84.55544, -14.232037) minor radius 0.000126 (-84.679446, -14.246565) -> (-84.88824, -14.270857) ccw
  line L374 (-84.88824, -14.270857) -> (-88.728395, -14.719187)
  line L375 (-88.024734, -12.120056) -> (-85.178358, -11.787747)
  ellipse E250 centre (-87.328667, -12.039046) end of major axis (-84.845558, -11.748928) minor radius 0.000126 (-84.845558, -11.748928) -> (-85.178358, -11.787747) ccw
  line L376 (-84.845558, -11.748928) -> (-84.55544, -14.232037)
  ellipse E251 centre (-85.781386, -14.375261) end of major axis (-86.571854, -14.467616) minor radius 0.000039 (-85.431798, -14.334452) -> (-85.431906, -14.334395) ccw
  line L377 (-87.96671, -12.616678) -> (-88.960362, -12.732685)
  line L378 (-103.934603, -8.925878) -> (-104.930437, -8.831506)
  line L379 (-107.736059, -8.063386) -> (-104.883255, -8.333737)
  ellipse E252 centre (-105.580746, -8.267694) end of major axis (-108.06959, -8.031786) minor radius 0.000028 (-107.736059, -8.063386) -> (-108.06959, -8.031786) ccw
  line L380 (-108.250451, -9.939885) -> (-108.06959, -8.031786)
  line L381 (-92.913465, -8.745042) -> (-93.001541, -8.730653)
  line L382 (-101.001541, -8.730653) -> (-101.089618, -8.745042)
  line L383 (-102.786101, -8.524436) -> (-102.001541, -8.396258)
  line L384 (-92.001541, -8.396258) -> (-91.216981, -8.524436)
  line L385 (-89.072645, -8.831506) -> (-90.068479, -8.925878)
  line L386 (-89.119827, -8.333737) -> (-86.267023, -8.063386)
  ellipse E253 centre (-88.422337, -8.267694) end of major axis (-85.933492, -8.031786) minor radius 0.000028 (-85.933492, -8.031786) -> (-86.266994, -8.063384) ccw
  line L387 (-85.933492, -8.031786) -> (-85.752631, -9.939885)
  spline S29 degree 3 poles (-103.277544, -7.946169) (-103.232654, -7.926359) (-103.143804, -7.887152) (-103.010994, -7.830981) (-102.880216, -7.777485) (-102.709894, -7.71057) (-102.501276, -7.632932) (-102.3337, -7.577853) (-102.251396, -7.550801) knots 0 0 0 0 0.13378969 0.26480564 0.39318317 0.51905417 0.76378306 1 1 1 1
  line L388 (-103.332626, -8.472633) -> (-103.277544, -7.946169)